Autodesk Fusion 360 part; units mm, degrees
(part 2 of 4)
sketch "SpaceBar Center" plane through (0, 17, 0) normal (0, 1, 0) x (-1, 0, 0)
  line L0 (-96.2371, 19.0203) -> (-96.2371, 18.4195)
  line L1 (-96.2371, 18.4195) -> (-95.4378, 18.4195)
  line L2 (-95.4378, 18.4195) -> (-95.4378, 5.6203)
  line L3 (-95.4378, 5.6203) -> (-96.2371, 5.6203)
  line L4 (-96.2371, 5.6203) -> (-96.2371, 5.0195)
  line L5 (-96.2371, 5.0195) -> (-110.23659, 5.0195)
  line L6 (-110.23659, 5.0195) -> (-110.23659, 5.6203)
  line L7 (-110.23659, 5.6203) -> (-111.03722, 5.6203)
  line L8 (-111.03722, 5.6203) -> (-111.03722, 18.4195)
  line L9 (-111.03722, 18.4195) -> (-110.23659, 18.4195)
  line L10 (-110.23659, 18.4195) -> (-110.23659, 19.0203)
  line L11 (-110.23659, 19.0203) -> (-96.2371, 19.0203)
  line L12 (-31.1441, 18.4195) -> (-31.1441, 5.6203)
  line L13 (-31.1441, 5.6203) -> (-31.9449, 5.6203)
  line L14 (-31.9449, 5.6203) -> (-31.9449, 5.0195)
  line L15 (-31.9449, 5.0195) -> (-45.9442, 5.0195)
  line L16 (-45.9442, 5.0195) -> (-45.9442, 5.6203)
  line L17 (-45.9442, 5.6203) -> (-46.745, 5.6203)
  line L18 (-46.745, 5.6203) -> (-46.745, 18.4195)
  line L19 (-46.745, 18.4195) -> (-45.9442, 18.4195)
  line L20 (-45.9442, 18.4195) -> (-45.9442, 19.0203)
  line L21 (-45.9442, 19.0203) -> (-31.9449, 19.0203)
  line L22 (-31.9449, 19.0203) -> (-31.9449, 18.4195)
  line L23 (-31.9449, 18.4195) -> (-31.1441, 18.4195)
  line L24 (-21.6191, 24.6704) -> (-22.4199, 24.6704)
  line L25 (-22.4199, 24.6704) -> (-22.4199, 24.0696)
  line L26 (-22.4199, 24.0696) -> (-36.4192, 24.0696)
  line L27 (-36.4192, 24.0696) -> (-36.4192, 24.6704)
  line L28 (-36.4192, 24.6704) -> (-37.2186, 24.6704)
  line L29 (-37.2186, 24.6704) -> (-37.2186, 37.4695)
  line L30 (-37.2186, 37.4695) -> (-36.4192, 37.4695)
  line L31 (-36.4192, 37.4695) -> (-36.4192, 38.0703)
  line L32 (-36.4192, 38.0703) -> (-22.4199, 38.0703)
  line L33 (-22.4199, 38.0703) -> (-22.4199, 37.4695)
  line L34 (-22.4199, 37.4695) -> (-21.6191, 37.4695)
  line L35 (-21.6191, 37.4695) -> (-21.6191, 24.6704)
  line L36 (-62.6115, -0.0297) -> (-46.391293, -0.0297)
  line L37 (-46.391293, -0.0297) -> (-46.391293, -0.6305)
  line L38 (-46.391293, -0.6305) -> (-45.592293, -0.6305)
  line L39 (-45.592293, -0.6305) -> (-45.592293, -3.205101)
  line L40 (-45.592293, -3.205101) -> (-43.156293, -3.205101)
  arc A0 (-43.156293, -8.205101) -> (-43.156293, -3.205101) centre (-43.156293, -5.705101) ccw
  line L41 (-43.156293, -8.205101) -> (-45.592293, -8.205101)
  line L42 (-45.592293, -8.205101) -> (-45.592293, -13.42971)
  line L43 (-45.592293, -13.42971) -> (-46.391293, -13.42971)
  line L44 (-46.391293, -13.42971) -> (-46.391293, -14.03054)
  line L45 (-46.391293, -14.03054) -> (-62.6115, -14.03054)
  line L46 (-62.6115, -14.03054) -> (-62.6115, -13.42971)
  line L47 (-62.6115, -13.42971) -> (-63.4123, -13.42971)
  line L48 (-63.4123, -13.42971) -> (-63.4123, -0.6305)
  line L49 (-63.4123, -0.6305) -> (-62.6115, -0.6305)
  line L50 (-62.6115, -0.6305) -> (-62.6115, -0.0297)
  circle A1 centre (-90.056293, 5.844899) radius 2.5
  line L51 (-100.2003, -13.42971) -> (-100.9996, -13.42971)
  line L52 (-100.9996, -13.42971) -> (-100.9996, -14.03054)
  line L53 (-100.9996, -14.03054) -> (-115.00047, -14.03054)
  line L54 (-115.00047, -14.03054) -> (-115.00047, -14)
  line L55 (-115.00047, -14) -> (-117.382293, -14)
  line L56 (-117.382293, -14) -> (-117.382293, -13.42971)
  line L57 (-117.382293, -13.42971) -> (-118.181293, -13.42971)
  line L58 (-118.181293, -13.42971) -> (-118.181293, -0.6305)
  line L59 (-118.181293, -0.6305) -> (-117.382293, -0.6305)
  line L60 (-117.382293, -0.6305) -> (-117.382293, -0.0297)
  line L61 (-117.382293, -0.0297) -> (-100.9996, -0.0297)
  line L62 (-100.9996, -0.0297) -> (-100.9996, -0.6305)
  line L63 (-100.9996, -0.6305) -> (-100.2003, -0.6305)
  line L64 (-100.2003, -0.6305) -> (-100.2003, -13.42971)
  line L65 (120.457, 5.6203) -> (120.457, 5.0195)
  line L66 (120.457, 5.0195) -> (106.457, 5.0195)
  line L67 (106.457, 5.0195) -> (106.457, 5.6203)
  line L68 (106.457, 5.6203) -> (105.656, 5.6203)
  line L69 (105.656, 5.6203) -> (105.656, 18.4195)
  line L70 (105.656, 18.4195) -> (106.457, 18.4195)
  line L71 (106.457, 18.4195) -> (106.457, 19.0203)
  line L72 (106.457, 19.0203) -> (120.457, 19.0203)
  line L73 (120.457, 19.0203) -> (120.457, 18.4195)
  line L74 (120.457, 18.4195) -> (121.257, 18.4195)
  line L75 (121.257, 18.4195) -> (121.257, 5.6203)
  line L76 (121.257, 5.6203) -> (120.457, 5.6203)
  circle A2 centre (62.431, -5.905101) radius 2.5
  line L77 (99.313, 57.1203) -> (113.313, 57.1203)
  line L78 (113.313, 57.1203) -> (113.313, 56.5195)
  line L79 (113.313, 56.5195) -> (114.112, 56.5195)
  line L80 (114.112, 56.5195) -> (114.112, 43.7204)
  line L81 (114.112, 43.7204) -> (113.313, 43.7204)
  line L82 (113.313, 43.7204) -> (113.313, 43.1196)
  line L83 (113.313, 43.1196) -> (99.313, 43.1196)
  line L84 (99.313, 43.1196) -> (99.313, 43.7204)
  line L85 (99.313, 43.7204) -> (98.513, 43.7204)
  line L86 (98.513, 43.7204) -> (98.513, 56.5195)
  line L87 (98.513, 56.5195) -> (99.313, 56.5195)
  line L88 (99.313, 56.5195) -> (99.313, 57.1203)
  line L89 (101.693, 24.0696) -> (101.693, 24.6704)
  line L90 (101.693, 24.6704) -> (100.894, 24.6704)
  line L91 (100.894, 24.6704) -> (100.894, 37.4695)
  line L92 (100.894, 37.4695) -> (101.693, 37.4695)
  line L93 (101.693, 37.4695) -> (101.693, 38.0703)
  line L94 (101.693, 38.0703) -> (115.694, 38.0703)
  line L95 (115.694, 38.0703) -> (115.694, 37.4695)
  line L96 (115.694, 37.4695) -> (116.493, 37.4695)
  line L97 (116.493, 37.4695) -> (116.493, 24.6704)
  line L98 (116.493, 24.6704) -> (115.694, 24.6704)
  line L99 (115.694, 24.6704) -> (115.694, 24.0696)
  line L100 (115.694, 24.0696) -> (101.693, 24.0696)
  line L101 (87.119, 56.5195) -> (87.918, 56.5195)
  line L102 (87.918, 56.5195) -> (87.918, 43.7204)
  line L103 (87.918, 43.7204) -> (87.119, 43.7204)
  line L104 (87.119, 43.7204) -> (87.119, 43.1196)
  line L105 (87.119, 43.1196) -> (73.118, 43.1196)
  line L106 (73.118, 43.1196) -> (73.118, 43.7204)
  line L107 (73.118, 43.7204) -> (72.319, 43.7204)
  line L108 (72.319, 43.7204) -> (72.319, 56.5195)
  line L109 (72.319, 56.5195) -> (73.118, 56.5195)
  line L110 (73.118, 56.5195) -> (73.118, 57.1203)
  line L111 (73.118, 57.1203) -> (87.119, 57.1203)
  line L112 (87.119, 57.1203) -> (87.119, 56.5195)
  line L113 (87.407, 5.0195) -> (87.407, 5.6203)
  line L114 (87.407, 5.6203) -> (86.606, 5.6203)
  line L115 (86.606, 5.6203) -> (86.606, 18.4195)
  line L116 (86.606, 18.4195) -> (87.407, 18.4195)
  line L117 (87.407, 18.4195) -> (87.407, 19.0203)
  line L118 (87.407, 19.0203) -> (101.407, 19.0203)
  line L119 (101.407, 19.0203) -> (101.407, 18.4195)
  line L120 (101.407, 18.4195) -> (102.207, 18.4195)
  line L121 (102.207, 18.4195) -> (102.207, 5.6203)
  line L122 (102.207, 5.6203) -> (101.407, 5.6203)
  line L123 (101.407, 5.6203) -> (101.407, 5.0195)
  line L124 (101.407, 5.0195) -> (87.407, 5.0195)
  line L125 (77.882, 24.6704) -> (77.081, 24.6704)
  line L126 (77.081, 24.6704) -> (77.081, 37.4695)
  line L127 (77.081, 37.4695) -> (77.882, 37.4695)
  line L128 (77.882, 37.4695) -> (77.882, 38.0703)
  line L129 (77.882, 38.0703) -> (91.882, 38.0703)
  line L130 (91.882, 38.0703) -> (91.882, 37.4695)
  line L131 (91.882, 37.4695) -> (92.682, 37.4695)
  line L132 (92.682, 37.4695) -> (92.682, 24.6704)
  line L133 (92.682, 24.6704) -> (91.882, 24.6704)
  line L134 (91.882, 24.6704) -> (91.882, 24.0696)
  line L135 (91.882, 24.0696) -> (77.882, 24.0696)
  line L136 (77.882, 24.0696) -> (77.882, 24.6704)
  circle A3 centre (90.731, 42.8948) radius 2.5
  line L137 (121.257, -0.6305) -> (121.257, -13.42971)
  line L138 (121.257, -13.42971) -> (120.457, -13.42971)
  line L139 (120.457, -13.42971) -> (120.457, -14.03054)
  line L140 (120.457, -14.03054) -> (106.457, -14.03054)
  line L141 (106.457, -14.03054) -> (106.457, -14)
  line L142 (106.457, -14) -> (101.407, -14)
  line L143 (101.407, -14) -> (101.407, -14.03054)
  line L144 (101.407, -14.03054) -> (87.407, -14.03054)
  line L145 (87.407, -14.03054) -> (87.407, -13.42971)
  line L146 (87.407, -13.42971) -> (86.606, -13.42971)
  line L147 (86.606, -13.42971) -> (86.606, -0.6305)
  line L148 (86.606, -0.6305) -> (87.407, -0.6305)
  line L149 (87.407, -0.6305) -> (87.407, -0.0297)
  line L150 (87.407, -0.0297) -> (120.457, -0.0297)
  line L151 (120.457, -0.0297) -> (120.457, -0.6305)
  line L152 (120.457, -0.6305) -> (121.257, -0.6305)
  line L153 (41.363, -0.6305) -> (42.162, -0.6305)
  line L154 (42.162, -0.6305) -> (42.162, -0.0297)
  line L155 (42.162, -0.0297) -> (58.544, -0.0297)
  line L156 (58.544, -0.0297) -> (58.544, -0.6305)
  line L157 (58.544, -0.6305) -> (59.343, -0.6305)
  line L158 (59.343, -0.6305) -> (59.343, -13.42971)
  line L159 (59.343, -13.42971) -> (58.544, -13.42971)
  line L160 (58.544, -13.42971) -> (58.544, -14.03054)
  line L161 (58.544, -14.03054) -> (44.543, -14.03054)
  line L162 (44.543, -14.03054) -> (44.543, -14)
  line L163 (44.543, -14) -> (42.162, -14)
  line L164 (42.162, -14) -> (42.162, -13.42971)
  line L165 (42.162, -13.42971) -> (41.363, -13.42971)
  line L166 (41.363, -13.42971) -> (41.363, -0.6305)
  line L167 (25.205, 18.4195) -> (26.006, 18.4195)
  line L168 (26.006, 18.4195) -> (26.006, 5.6203)
  line L169 (26.006, 5.6203) -> (25.205, 5.6203)
  line L170 (25.205, 5.6203) -> (25.205, 5.0195)
  line L171 (25.205, 5.0195) -> (11.206, 5.0195)
  line L172 (11.206, 5.0195) -> (11.206, 5.6203)
  line L173 (11.206, 5.6203) -> (10.405, 5.6203)
  line L174 (10.405, 5.6203) -> (10.405, 18.4195)
  line L175 (10.405, 18.4195) -> (11.206, 18.4195)
  line L176 (11.206, 18.4195) -> (11.206, 19.0203)
  line L177 (11.206, 19.0203) -> (17.022586, 19.0203)
  line L178 (17.022586, 19.0203) -> (17.022586, 19.279382)
  arc A4 (19.339414, 19.279382) -> (17.022586, 19.279382) centre (18.181, 21.4948) ccw
  line L179 (19.339414, 19.279382) -> (19.339414, 19.0203)
  line L180 (19.339414, 19.0203) -> (25.205, 19.0203)
  line L181 (25.205, 19.0203) -> (25.205, 18.4195)
  line L182 (-100.2003, 24.6704) -> (-100.9996, 24.6704)
  line L183 (-100.9996, 24.6704) -> (-100.9996, 24.0696)
  line L184 (-100.9996, 24.0696) -> (-115.00047, 24.0696)
  line L185 (-115.00047, 24.0696) -> (-115.00047, 24.6704)
  line L186 (-115.00047, 24.6704) -> (-115.79972, 24.6704)
  line L187 (-115.79972, 24.6704) -> (-115.79972, 37.4695)
  line L188 (-115.79972, 37.4695) -> (-115.00047, 37.4695)
  line L189 (-115.00047, 37.4695) -> (-115.00047, 38.0703)
  line L190 (-115.00047, 38.0703) -> (-100.9996, 38.0703)
  line L191 (-100.9996, 38.0703) -> (-100.9996, 37.4695)
  line L192 (-100.9996, 37.4695) -> (-100.2003, 37.4695)
  line L193 (-100.2003, 37.4695) -> (-100.2003, 24.6704)
  line L194 (-102.5816, 43.7204) -> (-103.3808, 43.7204)
  line L195 (-103.3808, 43.7204) -> (-103.3808, 43.1196)
  line L196 (-103.3808, 43.1196) -> (-117.38173, 43.1196)
  line L197 (-117.38173, 43.1196) -> (-117.38173, 43.7204)
  line L198 (-117.38173, 43.7204) -> (-118.18099, 43.7204)
  line L199 (-118.18099, 43.7204) -> (-118.18099, 56.5195)
  line L200 (-118.18099, 56.5195) -> (-117.38173, 56.5195)
  line L201 (-117.38173, 56.5195) -> (-117.38173, 57.1203)
  line L202 (-117.38173, 57.1203) -> (-103.3808, 57.1203)
  line L203 (-103.3808, 57.1203) -> (-103.3808, 56.5195)
  line L204 (-103.3808, 56.5195) -> (-102.5816, 56.5195)
  line L205 (-102.5816, 56.5195) -> (-102.5816, 43.7204)
  line L206 (-98.372293, -13.42971) -> (-99.171293, -13.42971)
  line L207 (-99.171293, -13.42971) -> (-99.171293, -0.6305)
  line L208 (-99.171293, -0.6305) -> (-98.372293, -0.6305)
  line L209 (-98.372293, -0.6305) -> (-98.372293, 0)
  line L210 (-98.372293, 0) -> (-65.401293, 0)
  line L211 (-65.401293, 0) -> (-65.401293, -0.6305)
  line L212 (-65.401293, -0.6305) -> (-64.602293, -0.6305)
  line L213 (-64.602293, -0.6305) -> (-64.602293, -13.42971)
  line L214 (-64.602293, -13.42971) -> (-65.401293, -13.42971)
  line L215 (-65.401293, -13.42971) -> (-65.401293, -14.03054)
  line L216 (-65.401293, -14.03054) -> (-98.372293, -14.03054)
  line L217 (-98.372293, -14.03054) -> (-98.372293, -13.42971)
  line L218 (-60.5185, 38.0703) -> (-60.5185, 37.4695)
  line L219 (-60.5185, 37.4695) -> (-59.7177, 37.4695)
  line L220 (-59.7177, 37.4695) -> (-59.7177, 24.6704)
  line L221 (-59.7177, 24.6704) -> (-60.5185, 24.6704)
  line L222 (-60.5185, 24.6704) -> (-60.5185, 24.0696)
  line L223 (-60.5185, 24.0696) -> (-74.5178, 24.0696)
  line L224 (-74.5178, 24.0696) -> (-74.5178, 24.6704)
  line L225 (-74.5178, 24.6704) -> (-75.3186, 24.6704)
  line L226 (-75.3186, 24.6704) -> (-75.3186, 37.4695)
  line L227 (-75.3186, 37.4695) -> (-74.5178, 37.4695)
  line L228 (-74.5178, 37.4695) -> (-74.5178, 38.0703)
  line L229 (-74.5178, 38.0703) -> (-60.5185, 38.0703)
  line L230 (-87.582873, 38.0703) -> (-79.5699, 38.0703)
  line L231 (-79.5699, 38.0703) -> (-79.5699, 37.4695)
  line L232 (-79.5699, 37.4695) -> (-78.7691, 37.4695)
  line L233 (-78.7691, 37.4695) -> (-78.7691, 24.6704)
  line L234 (-78.7691, 24.6704) -> (-79.5699, 24.6704)
  line L235 (-79.5699, 24.6704) -> (-79.5699, 24.0696)
  line L236 (-79.5699, 24.0696) -> (-93.5692, 24.0696)
  line L237 (-93.5692, 24.0696) -> (-93.5692, 24.6704)
  line L238 (-93.5692, 24.6704) -> (-94.3699, 24.6704)
  line L239 (-94.3699, 24.6704) -> (-94.3699, 37.4695)
  line L240 (-94.3699, 37.4695) -> (-93.5692, 37.4695)
  line L241 (-93.5692, 37.4695) -> (-93.5692, 38.0703)
  line L242 (-93.5692, 38.0703) -> (-89.429714, 38.0703)
  line L243 (-89.429714, 38.0703) -> (-89.429714, 38.271592)
  arc A5 (-89.429714, 42.918008) -> (-89.429714, 38.271592) centre (-88.506293, 40.5948) ccw
  line L244 (-89.429714, 42.918008) -> (-89.429714, 43.1196)
  line L245 (-89.429714, 43.1196) -> (-98.3317, 43.1196)
  line L246 (-98.3317, 43.1196) -> (-98.3317, 43.7204)
  line L247 (-98.3317, 43.7204) -> (-99.131, 43.7204)
  line L248 (-99.131, 43.7204) -> (-99.131, 56.5195)
  line L249 (-99.131, 56.5195) -> (-98.3317, 56.5195)
  line L250 (-98.3317, 56.5195) -> (-98.3317, 57.1203)
  line L251 (-98.3317, 57.1203) -> (-84.331, 57.1203)
  line L252 (-84.331, 57.1203) -> (-84.331, 56.5195)
  line L253 (-84.331, 56.5195) -> (-83.5316, 56.5195)
  line L254 (-83.5316, 56.5195) -> (-83.5316, 43.7204)
  line L255 (-83.5316, 43.7204) -> (-84.331, 43.7204)
  line L256 (-84.331, 43.7204) -> (-84.331, 43.1196)
  line L257 (-84.331, 43.1196) -> (-87.582873, 43.1196)
  line L258 (-87.582873, 43.1196) -> (-87.582873, 42.918008)
  arc A6 (-87.582873, 38.271592) -> (-87.582873, 42.918008) centre (-88.506293, 40.5948) ccw
  line L259 (-87.582873, 38.271592) -> (-87.582873, 38.0703)
  line L260 (-27.695, 5.6203) -> (-27.695, 18.4195)
  line L261 (-27.695, 18.4195) -> (-26.8942, 18.4195)
  line L262 (-26.8942, 18.4195) -> (-26.8942, 19.0203)
  line L263 (-26.8942, 19.0203) -> (-12.895, 19.0203)
  line L264 (-12.895, 19.0203) -> (-12.895, 18.4195)
  line L265 (-12.895, 18.4195) -> (-12.094, 18.4195)
  line L266 (-12.094, 18.4195) -> (-12.094, 5.6203)
  line L267 (-12.094, 5.6203) -> (-12.895, 5.6203)
  line L268 (-12.895, 5.6203) -> (-12.895, 5.0195)
  line L269 (-12.895, 5.0195) -> (-26.8942, 5.0195)
  line L270 (-26.8942, 5.0195) -> (-26.8942, 5.6203)
  line L271 (-26.8942, 5.6203) -> (-27.695, 5.6203)
  arc A7 (-13.437968, 42.823995) -> (-13.437968, 38.365605) centre (-12.306293, 40.5948) ccw
  line L272 (-13.437968, 42.823995) -> (-13.437968, 43.1196)
  line L273 (-13.437968, 43.1196) -> (-22.1317, 43.1196)
  line L274 (-22.1317, 43.1196) -> (-22.1317, 43.7204)
  line L275 (-22.1317, 43.7204) -> (-22.9311, 43.7204)
  line L276 (-22.9311, 43.7204) -> (-22.9311, 56.5195)
  line L277 (-22.9311, 56.5195) -> (-22.1317, 56.5195)
  line L278 (-22.1317, 56.5195) -> (-22.1317, 57.1203)
  line L279 (-22.1317, 57.1203) -> (-8.131, 57.1203)
  line L280 (-8.131, 57.1203) -> (-8.131, 56.5195)
  line L281 (-8.131, 56.5195) -> (-7.332, 56.5195)
  line L282 (-7.332, 56.5195) -> (-7.332, 43.7204)
  line L283 (-7.332, 43.7204) -> (-8.131, 43.7204)
  line L284 (-8.131, 43.7204) -> (-8.131, 43.1196)
  line L285 (-8.131, 43.1196) -> (-11.174619, 43.1196)
  line L286 (-11.174619, 43.1196) -> (-11.174619, 42.823995)
  arc A8 (-11.174619, 38.365605) -> (-11.174619, 42.823995) centre (-12.306293, 40.5948) ccw
  line L287 (-11.174619, 38.365605) -> (-11.174619, 38.0703)
  line L288 (-11.174619, 38.0703) -> (-3.37, 38.0703)
  line L289 (-3.37, 38.0703) -> (-3.37, 37.4695)
  line L290 (-3.37, 37.4695) -> (-2.569, 37.4695)
  line L291 (-2.569, 37.4695) -> (-2.569, 24.6704)
  line L292 (-2.569, 24.6704) -> (-3.37, 24.6704)
  line L293 (-3.37, 24.6704) -> (-3.37, 24.0696)
  line L294 (-3.37, 24.0696) -> (-17.369, 24.0696)
  line L295 (-17.369, 24.0696) -> (-17.369, 24.6704)
  line L296 (-17.369, 24.6704) -> (-18.17, 24.6704)
  line L297 (-18.17, 24.6704) -> (-18.17, 37.4695)
  line L298 (-18.17, 37.4695) -> (-17.369, 37.4695)
  line L299 (-17.369, 37.4695) -> (-17.369, 38.0703)
  line L300 (-17.369, 38.0703) -> (-13.437968, 38.0703)
  line L301 (-13.437968, 38.0703) -> (-13.437968, 38.365605)
  line L302 (68.069, 56.5195) -> (68.868, 56.5195)
  line L303 (68.868, 56.5195) -> (68.868, 43.7204)
  line L304 (68.868, 43.7204) -> (68.069, 43.7204)
  line L305 (68.069, 43.7204) -> (68.069, 43.1196)
  line L306 (68.069, 43.1196) -> (54.068, 43.1196)
  line L307 (54.068, 43.1196) -> (54.068, 43.7204)
  line L308 (54.068, 43.7204) -> (53.269, 43.7204)
  line L309 (53.269, 43.7204) -> (53.269, 56.5195)
  line L310 (53.269, 56.5195) -> (54.068, 56.5195)
  line L311 (54.068, 56.5195) -> (54.068, 57.1203)
  line L312 (54.068, 57.1203) -> (68.069, 57.1203)
  line L313 (68.069, 57.1203) -> (68.069, 56.5195)
  line L314 (67.556, -0.6305) -> (68.357, -0.6305)
  line L315 (68.357, -0.6305) -> (68.357, -0.0297)
  line L316 (68.357, -0.0297) -> (82.357, -0.0297)
  line L317 (82.357, -0.0297) -> (82.357, -0.6305)
  line L318 (82.357, -0.6305) -> (83.157, -0.6305)
  line L319 (83.157, -0.6305) -> (83.157, -13.42971)
  line L320 (83.157, -13.42971) -> (82.357, -13.42971)
  line L321 (82.357, -13.42971) -> (82.357, -14.03054)
  line L322 (82.357, -14.03054) -> (68.357, -14.03054)
  line L323 (68.357, -14.03054) -> (68.357, -13.42971)
  line L324 (68.357, -13.42971) -> (67.556, -13.42971)
  line L325 (67.556, -13.42971) -> (67.556, -0.6305)
  line L326 (68.357, 5.0195) -> (68.357, 5.6203)
  line L327 (68.357, 5.6203) -> (67.556, 5.6203)
  line L328 (67.556, 5.6203) -> (67.556, 18.4195)
  line L329 (67.556, 18.4195) -> (68.357, 18.4195)
  line L330 (68.357, 18.4195) -> (68.357, 19.0203)
  line L331 (68.357, 19.0203) -> (82.357, 19.0203)
  line L332 (82.357, 19.0203) -> (82.357, 18.4195)
  line L333 (82.357, 18.4195) -> (83.157, 18.4195)
  line L334 (83.157, 18.4195) -> (83.157, 5.6203)
  line L335 (83.157, 5.6203) -> (82.357, 5.6203)
  line L336 (82.357, 5.6203) -> (82.357, 5.0195)
  line L337 (82.357, 5.0195) -> (68.357, 5.0195)
  line L338 (-79.2817, 56.5195) -> (-79.2817, 57.1203)
  line L339 (-79.2817, 57.1203) -> (-65.281, 57.1203)
  line L340 (-65.281, 57.1203) -> (-65.281, 56.5195)
  line L341 (-65.281, 56.5195) -> (-64.4816, 56.5195)
  line L342 (-64.4816, 56.5195) -> (-64.4816, 43.7204)
  line L343 (-64.4816, 43.7204) -> (-65.281, 43.7204)
  line L344 (-65.281, 43.7204) -> (-65.281, 43.1196)
  line L345 (-65.281, 43.1196) -> (-79.2817, 43.1196)
  line L346 (-79.2817, 43.1196) -> (-79.2817, 43.7204)
  line L347 (-79.2817, 43.7204) -> (-80.0811, 43.7204)
  line L348 (-80.0811, 43.7204) -> (-80.0811, 56.5195)
  line L349 (-80.0811, 56.5195) -> (-79.2817, 56.5195)
  line L350 (-70.0449, 5.0195) -> (-84.0442, 5.0195)
  line L351 (-84.0442, 5.0195) -> (-84.0442, 5.6203)
  line L352 (-84.0442, 5.6203) -> (-84.8449, 5.6203)
  line L353 (-84.8449, 5.6203) -> (-84.8449, 18.4195)
  line L354 (-84.8449, 18.4195) -> (-84.0442, 18.4195)
  line L355 (-84.0442, 18.4195) -> (-84.0442, 19.0203)
  line L356 (-84.0442, 19.0203) -> (-70.0449, 19.0203)
  line L357 (-70.0449, 19.0203) -> (-70.0449, 18.4195)
  line L358 (-70.0449, 18.4195) -> (-69.2441, 18.4195)
  line L359 (-69.2441, 18.4195) -> (-69.2441, 5.6203)
  line L360 (-69.2441, 5.6203) -> (-70.0449, 5.6203)
  line L361 (-70.0449, 5.6203) -> (-70.0449, 5.0195)
  line L362 (-50.1941, 5.6203) -> (-50.9949, 5.6203)
  line L363 (-50.9949, 5.6203) -> (-50.9949, 5.0195)
  line L364 (-50.9949, 5.0195) -> (-64.9942, 5.0195)
  line L365 (-64.9942, 5.0195) -> (-64.9942, 5.6203)
  line L366 (-64.9942, 5.6203) -> (-65.795, 5.6203)
  line L367 (-65.795, 5.6203) -> (-65.795, 18.4195)
  line L368 (-65.795, 18.4195) -> (-64.9942, 18.4195)
  line L369 (-64.9942, 18.4195) -> (-64.9942, 19.0203)
  line L370 (-64.9942, 19.0203) -> (-50.9949, 19.0203)
  line L371 (-50.9949, 19.0203) -> (-50.9949, 18.4195)
  line L372 (-50.9949, 18.4195) -> (-50.1941, 18.4195)
  line L373 (-50.1941, 18.4195) -> (-50.1941, 5.6203)
  line L374 (35.532, 37.4695) -> (35.532, 24.6704)
  line L375 (35.532, 24.6704) -> (34.732, 24.6704)
  line L376 (34.732, 24.6704) -> (34.732, 24.0696)
  line L377 (34.732, 24.0696) -> (20.732, 24.0696)
  line L378 (20.732, 24.0696) -> (20.732, 24.6704)
  line L379 (20.732, 24.6704) -> (19.931, 24.6704)
  line L380 (19.931, 24.6704) -> (19.931, 37.4695)
  line L381 (19.931, 37.4695) -> (20.732, 37.4695)
  line L382 (20.732, 37.4695) -> (20.732, 38.0703)
  line L383 (20.732, 38.0703) -> (34.732, 38.0703)
  line L384 (34.732, 38.0703) -> (34.732, 37.4695)
  line L385 (34.732, 37.4695) -> (35.532, 37.4695)
  line L386 (15.682, 38.0703) -> (15.682, 37.4695)
  line L387 (15.682, 37.4695) -> (16.482, 37.4695)
  line L388 (16.482, 37.4695) -> (16.482, 24.6704)
  line L389 (16.482, 24.6704) -> (15.682, 24.6704)
  line L390 (15.682, 24.6704) -> (15.682, 24.0696)
  line L391 (15.682, 24.0696) -> (1.682, 24.0696)
  line L392 (1.682, 24.0696) -> (1.682, 24.6704)
  line L393 (1.682, 24.6704) -> (0.881, 24.6704)
  line L394 (0.881, 24.6704) -> (0.881, 37.4695)
  line L395 (0.881, 37.4695) -> (1.682, 37.4695)
  line L396 (1.682, 37.4695) -> (1.682, 38.0703)
  line L397 (1.682, 38.0703) -> (15.682, 38.0703)
  line L398 (-61.0311, 56.5195) -> (-60.2317, 56.5195)
  line L399 (-60.2317, 56.5195) -> (-60.2317, 57.1203)
  line L400 (-60.2317, 57.1203) -> (-46.231, 57.1203)
  line L401 (-46.231, 57.1203) -> (-46.231, 56.5195)
  line L402 (-46.231, 56.5195) -> (-45.4316, 56.5195)
  line L403 (-45.4316, 56.5195) -> (-45.4316, 43.7204)
  line L404 (-45.4316, 43.7204) -> (-46.231, 43.7204)
  line L405 (-46.231, 43.7204) -> (-46.231, 43.1196)
  line L406 (-46.231, 43.1196) -> (-60.2317, 43.1196)
  line L407 (-60.2317, 43.1196) -> (-60.2317, 43.7204)
  line L408 (-60.2317, 43.7204) -> (-61.0311, 43.7204)
  line L409 (-61.0311, 43.7204) -> (-61.0311, 56.5195)
  line L410 (10.919, 43.7204) -> (10.919, 43.1196)
  line L411 (10.919, 43.1196) -> (-3.082, 43.1196)
  line L412 (-3.082, 43.1196) -> (-3.082, 43.7204)
  line L413 (-3.082, 43.7204) -> (-3.881, 43.7204)
  line L414 (-3.881, 43.7204) -> (-3.881, 56.5195)
  line L415 (-3.881, 56.5195) -> (-3.082, 56.5195)
  line L416 (-3.082, 56.5195) -> (-3.082, 57.1203)
  line L417 (-3.082, 57.1203) -> (10.919, 57.1203)
  line L418 (10.919, 57.1203) -> (10.919, 56.5195)
  line L419 (10.919, 56.5195) -> (11.718, 56.5195)
  line L420 (11.718, 56.5195) -> (11.718, 43.7204)
  line L421 (11.718, 43.7204) -> (10.919, 43.7204)
  line L422 (26.782, -2.3007) -> (26.782, -1.3)
  line L423 (26.782, -1.3) -> (28.507, -1.3)
  line L424 (28.507, -1.3) -> (28.507, -0.1795)
  line L425 (28.507, -0.1795) -> (31.806, -0.1795)
  line L426 (31.806, -0.1795) -> (31.806, -1.3)
  line L427 (31.806, -1.3) -> (33.432, -1.3)
  line L428 (33.432, -1.3) -> (33.432, -4.7302)
  line L429 (33.432, -4.7302) -> (34.307, -4.7302)
  line L430 (34.307, -4.7302) -> (34.307, -7.53034)
  line L431 (34.307, -7.53034) -> (33.432, -7.53034)
  line L432 (33.432, -7.53034) -> (33.432, -14.0004)
  line L433 (33.432, -14.0004) -> (31.806, -14.0004)
  line L434 (31.806, -14.0004) -> (31.806, -14.78019)
  line L435 (31.806, -14.78019) -> (28.507, -14.78019)
  line L436 (28.507, -14.78019) -> (28.507, -14.0004)
  line L437 (28.507, -14.0004) -> (26.782, -14.0004)
  line L438 (26.782, -14.0004) -> (26.782, -12.99978)
  line L439 (26.782, -12.99978) -> (26.007, -12.99978)
  line L440 (26.007, -12.99978) -> (26.007, -13.42971)
  line L441 (26.007, -13.42971) -> (25.207, -13.42971)
  line L442 (25.207, -13.42971) -> (25.207, -14.03054)
  line L443 (25.207, -14.03054) -> (11.207, -14.03054)
  line L444 (11.207, -14.03054) -> (11.207, -13.42971)
  line L445 (11.207, -13.42971) -> (10.405, -13.42971)
  line L446 (10.405, -13.42971) -> (10.405, -12.99978)
  line L447 (10.405, -12.99978) -> (9.632, -12.99978)
  line L448 (9.632, -12.99978) -> (9.632, -14.0004)
  line L449 (9.632, -14.0004) -> (7.905, -14.0004)
  line L450 (7.905, -14.0004) -> (7.905, -14.78019)
  line L451 (7.905, -14.78019) -> (4.606, -14.78019)
  line L452 (4.606, -14.78019) -> (4.606, -14.0004)
  line L453 (4.606, -14.0004) -> (2.982, -14.0004)
  line L454 (2.982, -14.0004) -> (2.982, -7.53034)
  line L455 (2.982, -7.53034) -> (2.107, -7.53034)
  line L456 (2.107, -7.53034) -> (2.107, -4.7302)
  line L457 (2.107, -4.7302) -> (2.982, -4.7302)
  line L458 (2.982, -4.7302) -> (2.982, -1.3)
  line L459 (2.982, -1.3) -> (4.606, -1.3)
  line L460 (4.606, -1.3) -> (4.606, -0.1795)
  line L461 (4.606, -0.1795) -> (7.905, -0.1795)
  line L462 (7.905, -0.1795) -> (7.905, -1.3)
  line L463 (7.905, -1.3) -> (9.632, -1.3)
  line L464 (9.632, -1.3) -> (9.632, -2.3007)
  line L465 (9.632, -2.3007) -> (10.405, -2.3007)
  line L466 (10.405, -2.3007) -> (10.405, -0.6305)
  line L467 (10.405, -0.6305) -> (11.207, -0.6305)
  line L468 (11.207, -0.6305) -> (11.207, -0.0297)
  line L469 (11.207, -0.0297) -> (25.207, -0.0297)
  line L470 (25.207, -0.0297) -> (25.207, -0.6305)
  line L471 (25.207, -0.6305) -> (26.007, -0.6305)
  line L472 (26.007, -0.6305) -> (26.007, -2.3007)
  line L473 (26.007, -2.3007) -> (26.782, -2.3007)
  line L474 (-30.8506, -12.99978) -> (-30.8506, -14.0004)
  line L475 (-30.8506, -14.0004) -> (-32.576, -14.0004)
  line L476 (-32.576, -14.0004) -> (-32.576, -14.78019)
  line L477 (-32.576, -14.78019) -> (-35.8748, -14.78019)
  line L478 (-35.8748, -14.78019) -> (-35.8748, -14.0004)
  line L479 (-35.8748, -14.0004) -> (-37.4997, -14.0004)
  line L480 (-37.4997, -14.0004) -> (-37.4997, -7.53034)
  line L481 (-37.4997, -7.53034) -> (-38.3746, -7.53034)
  line L482 (-38.3746, -7.53034) -> (-38.3746, -4.7302)
  line L483 (-38.3746, -4.7302) -> (-37.4997, -4.7302)
  line L484 (-37.4997, -4.7302) -> (-37.4997, -1.3)
  line L485 (-37.4997, -1.3) -> (-35.8748, -1.3)
  line L486 (-35.8748, -1.3) -> (-35.8748, -0.1795)
  line L487 (-35.8748, -0.1795) -> (-32.576, -0.1795)
  line L488 (-32.576, -0.1795) -> (-32.576, -1.3)
  line L489 (-32.576, -1.3) -> (-30.8506, -1.3)
  line L490 (-30.8506, -1.3) -> (-30.8506, -2.3007)
  line L491 (-30.8506, -2.3007) -> (-30.0748, -2.3007)
  line L492 (-30.0748, -2.3007) -> (-30.0748, -0.6305)
  line L493 (-30.0748, -0.6305) -> (-29.2754, -0.6305)
  line L494 (-29.2754, -0.6305) -> (-29.2754, -0.0297)
  line L495 (-29.2754, -0.0297) -> (-15.275, -0.0297)
  line L496 (-15.275, -0.0297) -> (-15.275, -0.6305)
  line L497 (-15.275, -0.6305) -> (-14.475, -0.6305)
  line L498 (-14.475, -0.6305) -> (-14.475, -2.3007)
  line L499 (-14.475, -2.3007) -> (-13.701, -2.3007)
  line L500 (-13.701, -2.3007) -> (-13.701, -1.3)
  line L501 (-13.701, -1.3) -> (-11.976, -1.3)
  line L502 (-11.976, -1.3) -> (-11.976, -0.1795)
  line L503 (-11.976, -0.1795) -> (-8.675, -0.1795)
  line L504 (-8.675, -0.1795) -> (-8.675, -1.3)
  line L505 (-8.675, -1.3) -> (-7.05, -1.3)
  line L506 (-7.05, -1.3) -> (-7.05, -4.7302)
  line L507 (-7.05, -4.7302) -> (-6.176, -4.7302)
  line L508 (-6.176, -4.7302) -> (-6.176, -7.53034)
  line L509 (-6.176, -7.53034) -> (-7.05, -7.53034)
  line L510 (-7.05, -7.53034) -> (-7.05, -14.0004)
  line L511 (-7.05, -14.0004) -> (-8.675, -14.0004)
  line L512 (-8.675, -14.0004) -> (-8.675, -14.78019)
  line L513 (-8.675, -14.78019) -> (-11.976, -14.78019)
  line L514 (-11.976, -14.78019) -> (-11.976, -14.0004)
  line L515 (-11.976, -14.0004) -> (-13.701, -14.0004)
  line L516 (-13.701, -14.0004) -> (-13.701, -12.99978)
  line L517 (-13.701, -12.99978) -> (-14.475, -12.99978)
  line L518 (-14.475, -12.99978) -> (-14.475, -13.42971)
  line L519 (-14.475, -13.42971) -> (-15.275, -13.42971)
  line L520 (-15.275, -13.42971) -> (-15.275, -14.03054)
  line L521 (-15.275, -14.03054) -> (-29.2754, -14.03054)
  line L522 (-29.2754, -14.03054) -> (-29.2754, -13.42971)
  line L523 (-29.2754, -13.42971) -> (-30.0748, -13.42971)
  line L524 (-30.0748, -13.42971) -> (-30.0748, -12.99978)
  line L525 (-30.0748, -12.99978) -> (-30.8506, -12.99978)
  line L526 (-41.4685, 24.6704) -> (-41.4685, 24.0696)
  line L527 (-41.4685, 24.0696) -> (-55.4678, 24.0696)
  line L528 (-55.4678, 24.0696) -> (-55.4678, 24.6704)
  line L529 (-55.4678, 24.6704) -> (-56.2686, 24.6704)
  line L530 (-56.2686, 24.6704) -> (-56.2686, 37.4695)
  line L531 (-56.2686, 37.4695) -> (-55.4678, 37.4695)
  line L532 (-55.4678, 37.4695) -> (-55.4678, 38.0703)
  line L533 (-55.4678, 38.0703) -> (-41.4685, 38.0703)
  line L534 (-41.4685, 38.0703) -> (-41.4685, 37.4695)
  line L535 (-41.4685, 37.4695) -> (-40.6691, 37.4695)
  line L536 (-40.6691, 37.4695) -> (-40.6691, 24.6704)
  line L537 (-40.6691, 24.6704) -> (-41.4685, 24.6704)
  line L538 (49.019, 57.1203) -> (49.019, 56.5195)
  line L539 (49.019, 56.5195) -> (49.818, 56.5195)
  line L540 (49.818, 56.5195) -> (49.818, 43.7204)
  line L541 (49.818, 43.7204) -> (49.019, 43.7204)
  line L542 (49.019, 43.7204) -> (49.019, 43.1196)
  line L543 (49.019, 43.1196) -> (35.018, 43.1196)
  line L544 (35.018, 43.1196) -> (35.018, 43.7204)
  line L545 (35.018, 43.7204) -> (34.219, 43.7204)
  line L546 (34.219, 43.7204) -> (34.219, 56.5195)
  line L547 (34.219, 56.5195) -> (35.018, 56.5195)
  line L548 (35.018, 56.5195) -> (35.018, 57.1203)
  line L549 (35.018, 57.1203) -> (49.019, 57.1203)
  line L550 (15.968, 43.1196) -> (15.968, 43.7204)
  line L551 (15.968, 43.7204) -> (15.169, 43.7204)
  line L552 (15.169, 43.7204) -> (15.169, 56.5195)
  line L553 (15.169, 56.5195) -> (15.968, 56.5195)
  line L554 (15.968, 56.5195) -> (15.968, 57.1203)
  line L555 (15.968, 57.1203) -> (29.969, 57.1203)
  line L556 (29.969, 57.1203) -> (29.969, 56.5195)
  line L557 (29.969, 56.5195) -> (30.768, 56.5195)
  line L558 (30.768, 56.5195) -> (30.768, 43.7204)
  line L559 (30.768, 43.7204) -> (29.969, 43.7204)
  line L560 (29.969, 43.7204) -> (29.969, 43.1196)
  line L561 (29.969, 43.1196) -> (15.968, 43.1196)
  line L562 (-27.181, 43.1196) -> (-41.1817, 43.1196)
  line L563 (-41.1817, 43.1196) -> (-41.1817, 43.7204)
  line L564 (-41.1817, 43.7204) -> (-41.9811, 43.7204)
  line L565 (-41.9811, 43.7204) -> (-41.9811, 56.5195)
  line L566 (-41.9811, 56.5195) -> (-41.1817, 56.5195)
  line L567 (-41.1817, 56.5195) -> (-41.1817, 57.1203)
  line L568 (-41.1817, 57.1203) -> (-27.181, 57.1203)
  line L569 (-27.181, 57.1203) -> (-27.181, 56.5195)
  line L570 (-27.181, 56.5195) -> (-26.3816, 56.5195)
  line L571 (-26.3816, 56.5195) -> (-26.3816, 43.7204)
  line L572 (-26.3816, 43.7204) -> (-27.181, 43.7204)
  line L573 (-27.181, 43.7204) -> (-27.181, 43.1196)
  line L574 (45.057, 5.6203) -> (44.255, 5.6203)
  line L575 (44.255, 5.6203) -> (44.255, 5.0195)
  line L576 (44.255, 5.0195) -> (30.256, 5.0195)
  line L577 (30.256, 5.0195) -> (30.256, 5.6203)
  line L578 (30.256, 5.6203) -> (29.455, 5.6203)
  line L579 (29.455, 5.6203) -> (29.455, 18.4195)
  line L580 (29.455, 18.4195) -> (30.256, 18.4195)
  line L581 (30.256, 18.4195) -> (30.256, 19.0203)
  line L582 (30.256, 19.0203) -> (44.255, 19.0203)
  line L583 (44.255, 19.0203) -> (44.255, 18.4195)
  line L584 (44.255, 18.4195) -> (45.057, 18.4195)
  line L585 (45.057, 18.4195) -> (45.057, 5.6203)
  line L586 (-7.844, 19.0203) -> (6.155, 19.0203)
  line L587 (6.155, 19.0203) -> (6.155, 18.4195)
  line L588 (6.155, 18.4195) -> (6.956, 18.4195)
  line L589 (6.956, 18.4195) -> (6.956, 5.6203)
  line L590 (6.956, 5.6203) -> (6.155, 5.6203)
  line L591 (6.155, 5.6203) -> (6.155, 5.0195)
  line L592 (6.155, 5.0195) -> (-7.844, 5.0195)
  line L593 (-7.844, 5.0195) -> (-7.844, 5.6203)
  line L594 (-7.844, 5.6203) -> (-8.645, 5.6203)
  line L595 (-8.645, 5.6203) -> (-8.645, 18.4195)
  line L596 (-8.645, 18.4195) -> (-7.844, 18.4195)
  line L597 (-7.844, 18.4195) -> (-7.844, 19.0203)
  line L598 (58.031, 37.4695) -> (58.832, 37.4695)
  line L599 (58.832, 37.4695) -> (58.832, 38.0703)
  line L600 (58.832, 38.0703) -> (72.832, 38.0703)
  line L601 (72.832, 38.0703) -> (72.832, 37.4695)
  line L602 (72.832, 37.4695) -> (73.632, 37.4695)
  line L603 (73.632, 37.4695) -> (73.632, 24.6704)
  line L604 (73.632, 24.6704) -> (72.832, 24.6704)
  line L605 (72.832, 24.6704) -> (72.832, 24.0696)
  line L606 (72.832, 24.0696) -> (58.832, 24.0696)
  line L607 (58.832, 24.0696) -> (58.832, 24.6704)
  line L608 (58.832, 24.6704) -> (58.031, 24.6704)
  line L609 (58.031, 24.6704) -> (58.031, 37.4695)
  line L610 (38.981, 37.4695) -> (39.782, 37.4695)
  line L611 (39.782, 37.4695) -> (39.782, 38.0703)
  line L612 (39.782, 38.0703) -> (53.782, 38.0703)
  line L613 (53.782, 38.0703) -> (53.782, 37.4695)
  line L614 (53.782, 37.4695) -> (54.582, 37.4695)
  line L615 (54.582, 37.4695) -> (54.582, 24.6704)
  line L616 (54.582, 24.6704) -> (53.782, 24.6704)
  line L617 (53.782, 24.6704) -> (53.782, 24.0696)
  line L618 (53.782, 24.0696) -> (39.782, 24.0696)
  line L619 (39.782, 24.0696) -> (39.782, 24.6704)
  line L620 (39.782, 24.6704) -> (38.981, 24.6704)
  line L621 (38.981, 24.6704) -> (38.981, 37.4695)
  line L622 (63.307, 18.4195) -> (64.107, 18.4195)
  line L623 (64.107, 18.4195) -> (64.107, 5.6203)
  line L624 (64.107, 5.6203) -> (63.307, 5.6203)
  line L625 (63.307, 5.6203) -> (63.307, 5.0195)
  line L626 (63.307, 5.0195) -> (49.307, 5.0195)
  line L627 (49.307, 5.0195) -> (49.307, 5.6203)
  line L628 (49.307, 5.6203) -> (48.505, 5.6203)
  line L629 (48.505, 5.6203) -> (48.505, 18.4195)
  line L630 (48.505, 18.4195) -> (49.307, 18.4195)
  line L631 (49.307, 18.4195) -> (49.307, 19.0203)
  line L632 (49.307, 19.0203) -> (63.307, 19.0203)
  line L633 (63.307, 19.0203) -> (63.307, 18.4195)
  line L634 (-117.156293, -16.555101) -> (120.231, -16.555101)
  arc A9 (120.231, -16.555101) -> (123.231, -13.555101) centre (120.231, -13.555101) ccw
  line L635 (123.231, -13.555101) -> (123.231, 56.6448)
  arc A10 (123.231, 56.6448) -> (120.231, 59.6448) centre (120.231, 56.6448) ccw
  line L636 (120.231, 59.6448) -> (-117.156293, 59.6448)
  arc A11 (-117.156293, 59.6448) -> (-120.156293, 56.6448) centre (-117.156293, 56.6448) ccw
  line L637 (-120.156293, 56.6448) -> (-120.156293, -13.555101)
  arc A12 (-120.156293, -13.555101) -> (-117.156293, -16.555101) centre (-117.156293, -13.555101) ccw
  line L638 (2.107, -6.13027) -> (-6.176, -6.13027) construction
  line L639 (129.231, -22.555101) -> (-126.156293, -22.555101)
  line L640 (-2.0345, -6.13027) -> (-2.0345, -22.555101) construction
  constraint vertical L640
sketch "space_bar_cutout" plane through (0, 0, -22.555101) normal (0, 0, -1) x (-1, 0, 0)
  line L0 (-126.156293, 5) -> (129.231, 5)
  line L1 (129.231, 5) -> (129.231, 22)
  line L2 (129.231, 22) -> (-126.156293, 22)
  line L3 (-126.156293, 22) -> (-126.156293, 5)
  line L4 (-2.0345, 22) -> (-2.0345, 7) construction
  line L5 (-2.0345, 17.014854) -> (-44.571854, 17.014854)
  line L6 (-44.571854, 17.014854) -> (-44.571854, 22)
  line L7 (-2.0345, 17.014854) -> (40.502854, 17.014854)
  line L8 (40.502854, 17.014854) -> (40.502854, 22)
  arc A0 (-44.571854, 22) -> (-39.586708, 17.014854) centre (-39.586708, 22) ccw
  arc A1 (35.517708, 17.014854) -> (40.502854, 22) centre (35.517708, 22) ccw
  point P0 (-39.586708, 17.014854)
  point P1 (-6.176, 17)
  point P2 (2.107, 17)
  point P3 (-2.0345, 17)
  dimension "d18" = 4.985146
  dimension "d19" = 4.985146
  constraint perpendicular L4 L5
  constraint perpendicular L2 L6
  constraint perpendicular L4 L7
  constraint perpendicular L2 L8
  constraint equal L5 L7
  constraint tangent L5 A0
  constraint symmetric L4 A0 A1
  constraint coincident L4 P3
extrude "Extrude3" cut sketch "space_bar_cutout" against normal blind 4 contours L2 L5 L7 A0 A1 picked at (-2.0345, 20.338285) bodies 2
fillet "Fillet1" radius 1 2 edges at (44.571854, 22, -20.555101) (-40.502854, 22, -20.555101) on bodies 2
sketch "standoffs" plane through (0, 4, 0) normal (0, 1, 0) x (-1, 0, 0)
  line L0 (125.231, 61.6448) -> (-122.156293, 61.6448)
  line L1 (-122.156293, 61.6448) -> (-122.156293, -18.555101)
  line L2 (-122.156293, -18.555101) -> (125.231, -18.555101)
  line L3 (125.231, -18.555101) -> (125.231, 61.6448)
  arc A0 (19.339414, 19.279382) -> (17.022586, 19.279382) centre (18.181, 21.4948) ccw
  circle A1 centre (18.181, 21.4948) radius 2.5
  circle A2 centre (90.731, 42.8948) radius 2.5
  circle A3 centre (62.431, -5.905101) radius 2.5
  arc A4 (-13.437968, 42.823995) -> (-13.437968, 38.365605) centre (-12.306293, 40.5948) ccw
  arc A5 (-11.174619, 38.365605) -> (-11.174619, 42.823995) centre (-12.306293, 40.5948) ccw
  arc A6 (-87.582873, 38.271592) -> (-87.582873, 42.918008) centre (-88.506293, 40.5948) ccw
  arc A7 (-89.429714, 42.918008) -> (-89.429714, 38.271592) centre (-88.506293, 40.5948) ccw
  circle A8 centre (-90.056293, 5.844899) radius 2.5
  circle A9 centre (62.431, -5.905101) radius 2.5
  circle A10 centre (90.731, 42.8948) radius 2.5
  circle A11 centre (-12.306293, 40.5948) radius 2.5
  circle A12 centre (-90.056293, 5.844899) radius 2.5
  circle A13 centre (-88.506293, 40.5948) radius 2.5
  arc A14 (-43.156293, -8.205101) -> (-43.156293, -3.205101) centre (-43.156293, -5.705101) ccw
  circle A15 centre (-43.156293, -5.705101) radius 2.5
  constraint concentric A0 A1
  constraint concentric A3 A9
  constraint concentric A2 A10
  constraint concentric A5 A11
  constraint concentric A8 A12
  constraint concentric A6 A13
  constraint concentric A14 A15
extrude "Extrude4" add sketch "standoffs" along normal blind 5 contours A0 A1 | A2 A10 | A3 A9 | A4 A5 A11 | A6 A7 A13 | A8 A12 | A14 A15 picked at (19.886096, 21.041603) picked at (91.250575, 41.99487) picked at (62.344568, -6.465286) picked at (-12.788155, 39.914908) picked at (-87.893885, 41.159955) picked at (-89.751843, 6.372223) picked at (-42.442838, -4.950537) bodies 2
sketch "ref_for_holes" plane through (0, 9, 0) normal (0, 1, 0) x (-1, 0, 0)
  circle A0 centre (-12.306293, 40.5948) radius 2.5
  circle A1 centre (-43.156293, -5.705101) radius 2.5
  circle A2 centre (-88.506293, 40.5948) radius 2.5
  circle A3 centre (-90.056293, 5.844899) radius 2.5
  circle A4 centre (18.181, 21.4948) radius 2.5
  point P0 (-12.306293, 40.5948)
  point P1 (62.431, -5.905101)
  point P2 (90.731, 42.8948)
hole "Hole2" at (-18.181, 9, 21.4948) at (12.306293, 9, 40.5948) at (43.156293, 9, -5.705101) at (-62.431, 9, -5.905101) at (-90.731, 9, 42.8948) at (90.056293, 9, 5.844899) at (88.506293, 9, 40.5948) direction (0, -1, 0) diameter 1.875 depth 5 tip angle 180 bodies 2
thread "Thread2" "ISO Metric profile 2.3 M2.3x0.45 6H" major diameter 2.38 minor diameter 1.8754 pitch 0.45 angle 60 modelled right hand crest width 0.05625 on face at (-17.860356, 7.333333, 22.375762) crest through (-18.181, 9.253125, 22.4325) on face at (11.403833, 7.333333, 40.848713) crest through (12.306293, 9.253125, 41.5325) on face at (42.453374, 7.333333, -5.084771) crest through (43.156293, 9.253125, -4.767401) on face at (-63.13392, 7.333333, -5.284771) crest through (-62.431, 9.253125, -4.967401) on face at (-90.684269, 7.333333, 43.831135) crest through (-90.731, 9.253125, 43.8325) on face at (90.103024, 7.333333, 6.781234) crest through (90.056293, 9.253125, 6.782599) on face at (88.553024, 7.333333, 41.531135) crest through (88.506293, 9.253125, 41.5325) on bodies 2